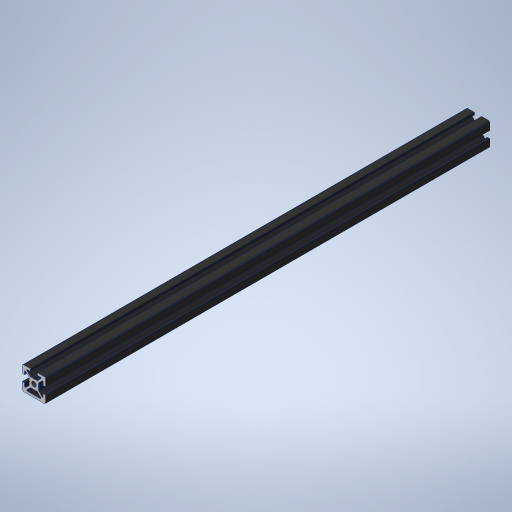
# Autodesk Inventor part: HFSFB5-2020-380
Saved by Autodesk Inventor 2024 (Build 280153000, 153)
## iProperties
Category: PARTsolutions
Company: MISUMI
Created: 2024-08-20
Part Number: HFSFB5-2020-380
Material: Aluminum 6061
Catalog Web Link: www.cadenas.de
Description: NFS5-2020, NFSB5-2020, HFS5-2020, HFSB5-2020, CAF5-2020, HFSY5-2020, NFSF5-2020, HFSF5-2020, HFSFB5-2020, NFST5-2020, HFST5-2020, HFSTB5-2020, HFSH5-2020, HFSC5-2020-HFS5 Series Aluminum Extrusions 20 Square -1 Slot-
Vendor: MISUMI
Document SubType Name: Modeling
Designer: psAdmin
Manufacturer: MISUMI
Mass: 230.97 g
Surface Area: 800.736 cm^2
Volume: 85.5443 cm^3
Density: 2.7 g/cm^3
Appearance: Aluminum - Flat
PSOL_IDENT_0: {$CADENAS_DATA/23d-libs/misumi/metric/38_al_extrusions_blackets/5/hfs5_2020.prj},680 {VTYP=3D},{NB=H
PSOL_IDENT_1: FSFB5-2020-440},{LINA=HFSFB5-2020-440},{NN=NFS5-2020, NFSB5-2020, HFS5-2020, HFSB5-2020, CAF5-2020,
PSOL_IDENT_2: HFSY5-2020, NFSF5-2020, HFSF5-2020, HFSFB5-2020, NFST5-2020, HFST5-2020, HFSTB5-2020, HFSH5-2020, HF
PSOL_IDENT_3: SC5-2020},{DATE=08.05.2023 08:39:06},{GEOMDATE=27.07.2021 03:20:00},{VERSION=},{LINEID=80},{WBVAR=L,
PSOL_IDENT_4: ALT1,ALT2,ALT4,ALT5,CP5,DL5,DR5,ALT6,ALT9,ALT10,ALT11,HP6,NHL6,DL6,NHR6,DR6,ALT7,ALT8,NH9,AH,BH,CH,D
PSOL_IDENT_5: H,EH,NH10,AV,BV,CV,DV,EV,NH11,AP,BP,CP,DP,EP,ALT12,ALT13,Z,NH12,XA,XB,XC,XD,XE,NH13,YA,YB,YC,YD,YE,A
PSOL_IDENT_6: LT16,HP16,DL16,DR16,ALT17,HQ17,JLP,ALT20},{WBNUMERIC=L,NH9,AH,BH,CH,DH,EH,NH10,AV,BV,CV,DV,EV,NH11,A
PSOL_IDENT_7: P,BP,CP,DP,EP,NH12,XA,XB,XC,XD,XE,NH13,YA,YB,YC,YD,YE,HQ17,JLP}  {NB=HFSFB5-2020-440},{LINA=HFSFB5-2
PSOL_IDENT_8: 020-440},{KT=DUMMY},{PN=HFSFB5-2020-440},{TPS=HFSFB5-2020},{MAT=A6N01SS-T5 Aluminum Alloy or 6005A-T
PSOL_IDENT_9: 5 Aluminum Alloy},{ST=Black Anodize},{FRMW=20},{FRMH=20},{FRD=4.2},{L=440},{MASS=0.53},{SA=195},{LX=
PSOL_IDENT_10: 0.834x10^4},{LY=0.746x10^4},{ALT1=},{M1=0},{DPL1=0},{DPR1=0},{ALT1PN=},{ALT2=},{ALT2ALG= '','w/o End
PSOL_IDENT_11: Tapping (Heli-Coil Insert)','LHP','with LHP (Tapping on the Left (Heli-Coil Insert))','RHP','with R
PSOL_IDENT_12: HP (Tapping on the Right (Heli-Coil Insert))','HPW','with HPW (Tapping on Both Ends (Heli-Coil Inser
PSOL_IDENT_13: t))' },{M2=0},{DP2=0},{ALT2PN=},{ALT4=},{ALT4ALG= '', 'w/o SC (High Precision Cut)', 'SC', 'with SC
PSOL_IDENT_14: (High Precision Cut)' },{ALT4PN=},{ALT5=},{ALT5ALG= '','w/o 45 Degree Cut','1','with 45 Degree Cut'
PSOL_IDENT_15: },{CP5=},{CP5ALG= '','N/A' },{DL5=},{DL5ALG= '','N/A' },{DR5=},{DR5ALG= '','N/A' },{FRMLALT5=0},{FRM
PSOL_IDENT_16: RALT5=0},{ALT5PN=},{ALT6=},{ALT6ALG= '','w/o Fastening Location Wrench Access Hole Alterations','1','
PSOL_IDENT_17: with Fastening Location Wrench Access Hole Alterations' },{ALT9=},{ALT9ALG= '','w/o Location Specifi
PSOL_IDENT_18: ed Wrench Access Hole Alteratons (Horizontal)','1','with Location Specified Wrench Access Hole Alter
PSOL_IDENT_19: atons (Horizontal)' },{ALT10=},{ALT10ALG= '','w/o Location Specified Wrench Access Hole Alteratons (
PSOL_IDENT_20: Vertical)','1','with Location Specified Wrench Access Hole Alteratons (Vertical)' },{ALT11=},{ALT11A
PSOL_IDENT_21: LG= '','w/o Location Specified Wrench Access Hole Alteratons (Crisscross)','1','with Location Specif
PSOL_IDENT_22: ied Wrench Access Hole Alteratons (Crisscross)' },{HP6=},{HP6ALG= '','N/A' },{NHL6=},{NHL6ALG= '','N
PSOL_IDENT_23: /A' },{DL6=},{DL6ALG= '','N/A' },{NHR6=},{NHR6ALG= '','N/A' },{DR6=},{DR6ALG= '','N/A' },{HL6=0.000}
PSOL_IDENT_24: ,{HL6D=0},{HR6=0.000},{HR6D=0},{J6=0},{J6D=0},{K6=0},{K6D=0},{DD6=0.00},{DD6ALG=0},{ALT7=},{ALT7ALG=
PSOL_IDENT_25: '','N/A' },{ALT8=},{ALT8ALG= '','N/A' },{ALT678PN=},{NH9=0},{NH9MAX=5},{NH9ALG=[0]},{AH=0.0},{AHMIN=
PSOL_IDENT_26: 7},{AHMAX=435},{AHALG=[0]},{BH=0.0},{BHMIN=2},{BHMAX=437},{BHALG=[0]},{CH=0.0},{CHMIN=2},{CHMAX=439}
PSOL_IDENT_27: ,{CHALG=[0]},{DH=0.0},{DHMIN=2},{DHMAX=441},{DHALG=[0]},{EH=0.0},{EHMIN=2},{EHMAX=433},{EHALG=[0]},{
PSOL_IDENT_28: NH10=0},{NH10MAX=5},{NH10ALG=[0]},{AV=0.0},{AVMIN=7},{AVMAX=435},{AVALG=[0]},{BV=0.0},{BVMIN=2},{BVM
PSOL_IDENT_29: AX=437},{BVALG=[0]},{CV=0.0},{CVMIN=2},{CVMAX=439},{CVALG=[0]},{DV=0.0},{DVMIN=2},{DVMAX=441},{DVALG=
PSOL_IDENT_30: [0]},{EV=0.0},{EVMIN=2},{EVMAX=433},{EVALG=[0]},{NH11=0},{NH11MAX=5},{NH11ALG=[0]},{AP=0.0},{APMIN=7
PSOL_IDENT_31: },{APMAX=435},{APALG=[0]},{BP=0.0},{BPMIN=2},{BPMAX=437},{BPALG=[0]},{CP=0.0},{CPMIN=2},{CPMAX=439},
PSOL_IDENT_32: {CPALG=[0]},{DP=0.0},{DPMIN=2},{DPMAX=441},{DPALG=[0]},{EP=0.0},{EPMIN=2},{EPMAX=433},{EPALG=[0]},{A
PSOL_IDENT_33: LT9PN=},{ALT10PN=},{ALT11PN=},{ALT91011PN=},{ALT12=},{ALT12ALG= '','w/o Counterbore Hole in Specifie
PSOL_IDENT_34: d Position (Vertical)','1','with Counterbore Hole in Specified Position (Vertical)' },{ALT13=},{ALT1
PSOL_IDENT_35: 3ALG= '','w/o Counterbore Hole in Specified Position (Horizontal)','1','with Counterbore Hole in Spe
PSOL_IDENT_36: cified Position (Horizontal)' },{Z=},{ZALG= '','N/A' },{DD12=0.0},{DD112=0.0},{NH12=0},{NH12MAX=5},{
PSOL_IDENT_37: NH12ALG=[0]},{XA=0.0},{XAMIN=7},{XAMAX=435},{XAALG=[0]},{XB=0.0},{XBMIN=2},{XBMAX=437},{XBALG=[0]},{
PSOL_IDENT_38: XC=0.0},{XCMIN=2},{XCMAX=439},{XCALG=[0]},{XD=0.0},{XDMIN=2},{XDMAX=441},{XDALG=[0]},{XE=0.0},{XEMIN=
PSOL_IDENT_39: 2},{XEMAX=433},{XEALG=[0]},{NH13=0},{NH13MAX=5},{NH13ALG=[0]},{YA=0.0},{YAMIN=7},{YAMAX=435},{YAALG=
PSOL_IDENT_40: [0]},{YB=0.0},{YBMIN=2},{YBMAX=437},{YBALG=[0]},{YC=0.0},{YCMIN=2},{YCMAX=439},{YCALG=[0]},{YD=0.0},
PSOL_IDENT_41: {YDMIN=2},{YDMAX=441},{YDALG=[0]},{YE=0.0},{YEMIN=2},{YEMAX=433},{YEALG=[0]},{ALT12PN=},{ALT13PN=},{
PSOL_IDENT_42: ALT1213PN=},{ALT16=},{ALT16ALG= '','w/o M Type Hole Alteration','1','with M Type Hole Alteration' },
PSOL_IDENT_43: {HP16=},{HP16ALG= '','N/A' },{DL16=},{DL16ALG= '','N/A' },{DR16=},{DR16ALG= '','N/A' },{H116=0},{D16=
PSOL_IDENT_44: 0.0},{ALT16PN=},{ALT17=},{ALT17ALG= '','w/o L Type Hole Alteration (Top)','1','with L Type Hole Alte
PSOL_IDENT_45: ration (Top)' },{HQ17=0},{HQ17ALG=0},{JLP=0},{JLPMIN=4.9},{JLPMAX=0},{JLPALG=[0]},{L17=0},{D17=0.0},
PSOL_IDENT_46: {ALT17PN=},{ALT20=},{ALT20PN=},{ERRORALT01=OK},{ERRORALT02=OK},{ERRORALT05=OK},{ERRORALT06091=OK},{E
PSOL_IDENT_47: RRORALT06092=OK},{ERRORALT06093=OK},{ERRORALT06094=OK},{ERRORALT06101=OK},{ERRORALT06102=OK},{ERRORA
PSOL_IDENT_48: LT06103=OK},{ERRORALT06104=OK},{ERRORALT06111=OK},{ERRORALT06112=OK},{ERRORALT06113=OK},{ERRORALT061
PSOL_IDENT_49: 14=OK},{ERRORALT06121=OK},{ERRORALT06122=OK},{ERRORALT06123=OK},{ERRORALT06124=OK},{ERRORALT06131=OK
PSOL_IDENT_50: },{ERRORALT06132=OK},{ERRORALT06133=OK},{ERRORALT06134=OK},{ERRORALT0616=OK},{ERRORALT06171=OK},{ERR
PSOL_IDENT_51: ORALT06172=OK},{ERRORALT06173=OK},{ERRORALT0911=OK},{ERRORALT0913=OK},{ERRORALT0916=OK},{ERRORALT091
PSOL_IDENT_52: 7=OK},{ERRORALT1011=OK},{ERRORALT1012=OK},{ERRORALT1016=OK},{ERRORALT1017=OK},{ERRORALT1112=OK},{ERR
PSOL_IDENT_53: ORALT1113=OK},{ERRORALT1116=OK},{ERRORALT1117=OK},{ERRORALT1216=OK},{ERRORALT1217=OK},{ERRORALT1316=
PSOL_IDENT_54: OK},{ERRORALT1317=OK},{ERRORALT1617=OK},{ERRORPN=},{TFW=0}
NB: HFSFB5-2020-440
NN: NFS5-2020, NFSB5-2020, HFS5-2020, HFSB5-2020, CAF5-2020, HFSY5-2020, NFSF5-2020, HFSF5-2020, HFSFB5-2020, NFST5-2020, HFST5-2020, HFSTB5-2020, HFSH5-2020, HFSC5-2020
NT: HFS5 Series Aluminum Extrusions 20 Square -1 Slot-
NBSYN: $PN.
LINA: HFSFB5-2020-440
CATALOG: Misumi
PN: HFSFB5-2020-440
TPS: HFSFB5-2020
MAT: A6N01SS-T5 Aluminum Alloy or 6005A-T5 Aluminum Alloy
ST: Black Anodize
L: 440
MASS: 0.53
SA: 195
LX: 0.834x10^4
LY: 0.746x10^4
ALT1: w/o End Tapping
M1: 0
DPL1: 0
DPR1: 0
ALT2: w/o End Tapping (Heli-Coil Insert)
M2: 0
DP2: 0
ALT4: w/o SC (High Precision Cut)
ALT5: w/o 45 Degree Cut
CP5: N/A
DL5: N/A
DR5: N/A
ALT6: w/o Fastening Location Wrench Access Hole Alterations
ALT9: w/o Location Specified Wrench Access Hole Alteratons (Horizontal)
ALT10: w/o Location Specified Wrench Access Hole Alteratons (Vertical)
ALT11: w/o Location Specified Wrench Access Hole Alteratons (Crisscross)
HP6: N/A
NHL6: N/A
DL6: N/A
NHR6: N/A
DR6: N/A
HL6D: 0
HR6D: 0
J6D: 0
K6D: 0
DD6: 0
ALT7: N/A
ALT8: N/A
NH9: 0
AH: 0
BH: 0
CH: 0
DH: 0
EH: 0
NH10: 0
AV: 0
BV: 0
CV: 0
DV: 0
EV: 0
NH11: 0
AP: 0
BP: 0
CP: 0
DP: 0
EP: 0
ALT12: w/o Counterbore Hole in Specified Position (Vertical)
ALT13: w/o Counterbore Hole in Specified Position (Horizontal)
Z: N/A
DD12: 0
DD112: 0
NH12: 0
XA: 0
XB: 0
XC: 0
XD: 0
XE: 0
NH13: 0
YA: 0
YB: 0
YC: 0
YD: 0
YE: 0
ALT16: w/o M Type Hole Alteration
HP16: N/A
DL16: N/A
DR16: N/A
H116: 0
D16: 0
ALT17: w/o L Type Hole Alteration (Top)
HQ17: 0
JLP: 0
D17: 0
ALT20: w/o CW (End Face C Chamfering)
SUPPLIER: MISUMI
ARTICLENO: HFSFB5-2020-440
BOMINFO: HFSFB5-2020-440
CREATOR: CADENAS GmbH
Title: HFSFB5-2020-440
Author: Cadenas PARTsolutions
Comments: HFS5 Series Aluminum Extrusions 20 Square -1 Slot-
Autodesk Inventor part; units mm, degrees
sketch "Sketch_63" plane through (0, 0, 0) normal (0, 0, 1) x (1, 0, 0)
  line L0 (-10, -3) -> (-10, -9)
  arc A0 (-10, -9) -> (-9, -10) centre (-9, -9) ccw
  line L1 (-9, -10) -> (9, -10)
  arc A1 (9, -10) -> (10, -9) centre (9, -9) ccw
  line L2 (10, -9) -> (10, -3)
  line L3 (10, -3) -> (8, -3)
  line L4 (8, -3) -> (8, -6)
  line L5 (8, -6) -> (7.0607, -6)
  line L6 (7.0607, -6) -> (4, -2.9393)
  line L7 (4, -2.9393) -> (4, -0.5196)
  line L8 (4, -0.5196) -> (3.7, 0)
  line L9 (3.7, 0) -> (4, 0.5196)
  line L10 (4, 0.5196) -> (4, 2.9393)
  line L11 (4, 2.9393) -> (7.0607, 6)
  line L12 (7.0607, 6) -> (8, 6)
  line L13 (8, 6) -> (8, 3)
  line L14 (8, 3) -> (10, 3)
  line L15 (10, 3) -> (10, 9)
  arc A2 (10, 9) -> (9, 10) centre (9, 9) ccw
  line L16 (9, 10) -> (3, 10)
  line L17 (3, 10) -> (3, 8)
  line L18 (3, 8) -> (6, 8)
  line L19 (6, 8) -> (6, 7.0607)
  line L20 (6, 7.0607) -> (2.9393, 4)
  line L21 (2.9393, 4) -> (0.5196, 4)
  line L22 (0.5196, 4) -> (0, 3.7)
  line L23 (0, 3.7) -> (-0.5196, 4)
  line L24 (-0.5196, 4) -> (-2.9393, 4)
  line L25 (-2.9393, 4) -> (-6, 7.0607)
  line L26 (-6, 7.0607) -> (-6, 8)
  line L27 (-6, 8) -> (-3, 8)
  line L28 (-3, 8) -> (-3, 10)
  line L29 (-3, 10) -> (-9, 10)
  arc A3 (-9, 10) -> (-10, 9) centre (-9, 9) ccw
  line L30 (-10, 9) -> (-10, 3)
  line L31 (-10, 3) -> (-8, 3)
  line L32 (-8, 3) -> (-8, 6)
  line L33 (-8, 6) -> (-7.0607, 6)
  line L34 (-7.0607, 6) -> (-4, 2.9393)
  line L35 (-4, 2.9393) -> (-4, 0.5196)
  line L36 (-4, 0.5196) -> (-3.7, 0)
  line L37 (-3.7, 0) -> (-4, -0.5196)
  line L38 (-4, -0.5196) -> (-4, -2.9393)
  line L39 (-4, -2.9393) -> (-7.0607, -6)
  line L40 (-7.0607, -6) -> (-8, -6)
  line L41 (-8, -6) -> (-8, -3)
  line L42 (-8, -3) -> (-10, -3)
  line L43 (-6, -7.2678) -> (-6, -7.5)
  arc A4 (-6, -7.5) -> (-5.5, -8) centre (-5.5, -7.5) ccw
  line L44 (-5.5, -8) -> (5.5, -8)
  arc A5 (5.5, -8) -> (6, -7.5) centre (5.5, -7.5) ccw
  line L45 (6, -7.5) -> (6, -7.2678)
  arc A6 (6, -7.2678) -> (5.8536, -6.9142) centre (5.5, -7.2678) ccw
  line L46 (5.8536, -6.9142) -> (3.0858, -4.1464)
  arc A7 (3.0858, -4.1464) -> (2.7322, -4) centre (2.7322, -4.5) ccw
  line L47 (2.7322, -4) -> (-2.7322, -4)
  arc A8 (-2.7322, -4) -> (-3.0858, -4.1464) centre (-2.7322, -4.5) ccw
  line L48 (-3.0858, -4.1464) -> (-5.8536, -6.9142)
  arc A9 (-5.8536, -6.9142) -> (-6, -7.2678) centre (-5.5, -7.2678) ccw
  constraints: 98 end point, 20 point on circle, 10 centre point
extrude "Extrusion1" add sketch "Sketch_63" along normal mid plane 380
sketch "Sketch2" plane through (0, 0, 190) normal (0, 0, 1) x (-1, 0, 0)
  point P0 (0, 0)
hole "Hole1" at (0, 0, 190) direction (0, 0, -1) diameter 4.2 depth 440
ref_plane "C1_XY" through (0, 0, 0) normal (0, 0, 1) x (1, 0, 0)
ref_plane "C1_YZ" through (0, 0, 0) normal (1, 0, 0) x (0, 1, 0)
ref_plane "C1_ZX" through (0, 0, 0) normal (0, 1, 0) x (0, 0, 1)
thread "Thread1" size "M5x0.8" class "6H" standard "ANSI Metric M Profile" length 10
thread "Thread2" size "M5x0.8" class "6H" standard "ANSI Metric M Profile" length 10
body "Solid1"
